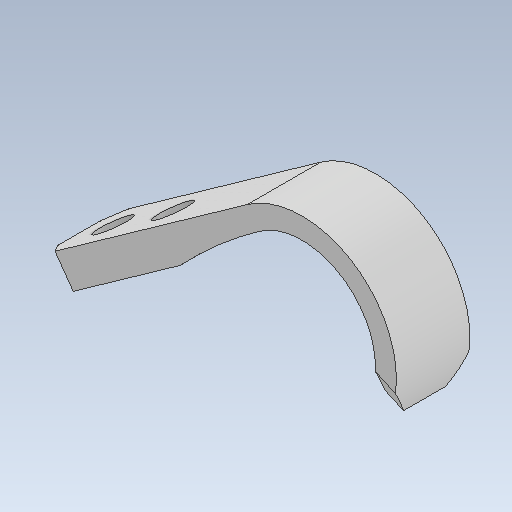
# Autodesk Inventor part: foot_2
Saved by Autodesk Inventor 2023 (Build 270158000, 158)
## iProperties
Created: 2020-12-13
Part Number: foot_2
Material: Generic
Document SubType Name: Modeling
Designer: Shuang Peng
Density: 1 g/cm^3
Appearance: Default
Author: Shuang Peng
Autodesk Inventor part; units mm, degrees
ref_plane "YZ Plane" through (0, 0, 0) normal (1, 0, 0) x (0, 1, 0)
ref_plane "XZ Plane" through (0, 0, 0) normal (0, 1, 0) x (-1, 0, 0)
sketch "Sketch1" plane through (0, 0, 0) normal (0, 0, 1) x (1, 0, 0)
  line L0 (24.6201, 20.01) -> (22.9897, 18.8516) projected
  line L1 (22.9897, 18.8516) -> (25.0169, 15.9984) projected
  line L2 (25.0169, 15.9984) -> (26.6472, 17.1568) projected
  line L3 (26.6472, 17.1568) -> (24.6201, 20.01) projected
  circle A0 centre (-21.6472, -15.01) radius 3.075 projected
  circle A1 centre (9.3299, 6.9995) radius 3.075 projected
  line L4 (22.9897, 18.8516) -> (25.0169, 15.9984) projected
  line L5 (22.9897, 18.8516) -> (13.1347, 11.8496) projected
  arc A2 (11.2202, 11.6284) -> (13.1347, 11.8496) centre (11.9763, 13.4799) ccw projected
  arc A3 (11.2202, 11.6284) -> (4.3368, 6.7377) centre (9.3299, 6.9995) ccw projected
  arc A4 (3.4979, 5.0025) -> (4.3368, 6.7377) centre (2.3395, 6.6329) ccw projected
  line L6 (3.4979, 5.0025) -> (-17.8424, -10.1599) projected
  arc A5 (-19.7569, -10.3811) -> (-17.8424, -10.1599) centre (-19.0008, -8.5295) ccw projected
  arc A6 (-19.7569, -10.3811) -> (-16.6541, -14.7482) centre (-21.6472, -15.01) ccw projected
  arc A7 (-15.8152, -13.0131) -> (-16.6541, -14.7482) centre (-14.6569, -14.6434) ccw projected
  line L7 (-15.8152, -13.0131) -> (5.5251, 2.1494) projected
  arc A8 (7.4396, 2.3706) -> (5.5251, 2.1494) centre (6.6835, 0.519) ccw projected
  arc A9 (7.4396, 2.3706) -> (14.323, 7.2613) centre (9.3299, 6.9995) ccw projected
  arc A10 (15.1619, 8.9964) -> (14.323, 7.2613) centre (16.3203, 7.366) ccw projected
  line L8 (15.1619, 8.9964) -> (25.0169, 15.9984) projected
  line L9 (17.6802, 10.7857) -> (15.653, 13.6388)
  line L10 (15.653, 13.6388) -> (13.2074, 11.9012)
  line L11 (13.2074, 11.9012) -> (11.4698, 14.3468)
  line L12 (11.4698, 14.3468) -> (31.0343, 28.2475)
  line L13 (31.0343, 28.2475) -> (41.4599, 13.5741)
  arc A11 (41.4599, 13.5741) -> (31.0343, 28.2475) centre (36.2471, 20.9108) ccw
  line L14 (41.4599, 13.5741) -> (40.3015, 15.2045)
  line L15 (40.3015, 15.2045) -> (32.1927, 26.6171)
  arc A12 (40.3015, 15.2045) -> (32.1927, 26.6171) centre (36.2471, 20.9108) ccw
  line L16 (15.653, 13.6388) -> (32.7719, 25.802)
  arc A13 (32.1927, 26.6171) -> (24.6201, 20.01) centre (61.4422, -14.5498) ccw
  point P0 (0, 0)
  dimension "d0" = 3
  dimension "d1" = 3
  dimension "d2" = 24
  dimension "d3" = 18
  dimension "d4" = 9
  dimension "d5" = 2
  dimension "d6" = 14
  dimension "d7" = 7
  constraints: 16 end point, 6 point on circle, 4 perpendicular, 4 point on line, 3 centre point, 1 line through centre, 3 other
  measures "d0" distance of L9.end L10.end
  measures "d1" distance of L10.end L11.end
  measures "d2" distance of L11.end L12.end
  measures "d3" distance of L12.end L13.end
  measures "d4" radius of A11
  measures "d5" distance of L13.end L14.end
  measures "d6" distance of L14.end L15.end
  measures "d7" radius of A12
ref_plane "Work Plane1" through (-46.048, -45.8021, -7) normal (0, 0, -1) x (0, 1, 0)
extrude "Extrusion1" add sketch "Sketch1" against normal up to surface (7 mm away) contours L0 L5 L11 L12 L13 A13 | L13 A11 A12
sketch "Sketch2" plane through (11.4698, 14.3468, 0) normal (-0.5791965, 0.8151879, 0) x (0.8151879, 0.5791965, 0)
  circle A0 centre (4, 3.5) radius 1 projected
  circle A1 centre (11, 3.5) radius 1 projected
  circle A2 centre (4, 3.5) radius 1.6
  circle A3 centre (11, 3.5) radius 1.6
  point P0 (-17.6597, 0)
  dimension "d10" = 3.2
  dimension "d11" = 3.2
  constraints: 2 centre point, 2 coincident
  measures "d10" diameter of A2
  measures "d11" diameter of A3
extrude "Extrusion2" cut sketch "Sketch2" against normal blind 10 contours A0 | A1 | A2 | A3
chamfer "Chamfer1" distance 1.5 angle 45 2 edges at (12.3386, 13.124, 0) (12.3386, 13.124, -7)
sketch "Sketch3" plane through (0, 0, 0) normal (0, 0, 1) x (1, 0, 0)
  line L0 (14.4302, 12.77) -> (12.6926, 15.2156) projected
  line L1 (14.4302, 12.77) -> (24.6201, 20.01) projected
  arc A0 (32.1927, 26.6171) -> (24.6201, 20.01) centre (61.4422, -14.5498) ccw projected
  arc A1 (40.3015, 15.2045) -> (32.1927, 26.6171) centre (36.2471, 20.9108) ccw projected
  line L2 (40.3015, 15.2045) -> (41.4599, 13.5741) projected
  arc A2 (41.4599, 13.5741) -> (31.0343, 28.2475) centre (36.2471, 20.9108) ccw projected
  line L3 (31.0343, 28.2475) -> (12.6926, 15.2156) projected
  line L4 (36.2471, 20.9108) -> (44.4299, 17.1634)
  point P0 (0, 0)
  point P1 (42.6115, 17.9962)
  dimension "d17" = 30
  constraints: 2 end point, 1 point on circle
  measures "d17" angle of L2 L4
extrude "Extrusion3" cut sketch "Sketch3" against normal blind 10 contours A2 L2 A1 L4
chamfer "Chamfer2" distance 1.5 angle 60 2 edges at (43.5207, 17.5798, 0) (43.5207, 17.5798, -7) measured on face at (43.5207, 17.5798, -6.5) measured on face at (43.5207, 17.5798, -0.5)
body "Solid1"
